Autodesk Inventor part; units mm, degrees
(part 2 of 3)
  line L886 (-89.9741, -91.3777) -> (-89.3883, -91.9634) construction
  line L887 (-89.3883, -91.9634) -> (-88.4384, -91.9634) construction
  line L888 (-88.4384, -91.9634) -> (-87.8528, -91.3777) construction
  line L889 (-87.8528, -91.3777) -> (-82.9029, -86.4278)
  spline S5 degree 3 poles (-82.9029, -86.4278) (-82.3172, -85.8421) (-82.3172, -84.8923) (-82.9029, -84.3067) knots 4 4 4 4 5 5 5 5
  line L890 (-82.9029, -86.4278) -> (-82.3172, -85.8421) construction
  line L891 (-82.3172, -85.8421) -> (-82.3172, -84.8923) construction
  line L892 (-82.3172, -84.8923) -> (-82.9029, -84.3067) construction
  line L893 (-82.9029, -84.3067) -> (-84.3171, -82.8924)
  spline S6 degree 3 poles (-84.3171, -82.8924) (-84.9029, -82.3064) (-85.8527, -82.3064) (-86.4384, -82.8924) knots 6 6 6 6 7 7 7 7
  line L894 (-84.3171, -82.8924) -> (-84.9029, -82.3064) construction
  line L895 (-84.9029, -82.3064) -> (-85.8527, -82.3064) construction
  line L896 (-85.8527, -82.3064) -> (-86.4384, -82.8924) construction
  line L897 (-86.4384, -82.8924) -> (-91.3883, -87.842)
  spline S7 degree 3 poles (-72.0243, -68.4782) (-72.6101, -69.0638) (-72.6101, -70.0136) (-72.0243, -70.5993) knots 0 0 0 0 1 1 1 1
  line L898 (-72.0243, -68.4782) -> (-72.6101, -69.0638) construction
  line L899 (-72.6101, -69.0638) -> (-72.6101, -70.0136) construction
  line L900 (-72.6101, -70.0136) -> (-72.0243, -70.5993) construction
  line L901 (-72.0243, -70.5993) -> (-70.6101, -72.0135)
  spline S8 degree 3 poles (-70.6101, -72.0135) (-70.0242, -72.5995) (-69.0746, -72.5995) (-68.4888, -72.0135) knots 2 2 2 2 3 3 3 3
  line L902 (-70.6101, -72.0135) -> (-70.0242, -72.5995) construction
  line L903 (-70.0242, -72.5995) -> (-69.0746, -72.5995) construction
  line L904 (-69.0746, -72.5995) -> (-68.4888, -72.0135) construction
  line L905 (-68.4888, -72.0135) -> (-63.539, -67.064)
  spline S9 degree 3 poles (-63.539, -67.064) (-62.9532, -66.4779) (-62.9532, -65.5285) (-63.539, -64.9425) knots 4 4 4 4 5 5 5 5
  line L906 (-63.539, -67.064) -> (-62.9532, -66.4779) construction
  line L907 (-62.9532, -66.4779) -> (-62.9532, -65.5285) construction
  line L908 (-62.9532, -65.5285) -> (-63.539, -64.9425) construction
  line L909 (-63.539, -64.9425) -> (-64.9532, -63.5282)
  spline S10 degree 3 poles (-64.9532, -63.5282) (-65.5391, -62.9426) (-66.4887, -62.9426) (-67.0745, -63.5282) knots 6 6 6 6 7 7 7 7
  line L910 (-64.9532, -63.5282) -> (-65.5391, -62.9426) construction
  line L911 (-65.5391, -62.9426) -> (-66.4887, -62.9426) construction
  line L912 (-66.4887, -62.9426) -> (-67.0745, -63.5282) construction
  line L913 (-67.0745, -63.5282) -> (-72.0243, -68.4782)
  spline S11 degree 3 poles (-52.6603, -49.114) (-53.2461, -49.7) (-53.2461, -50.6498) (-52.6603, -51.2355) knots 0 0 0 0 1 1 1 1
  line L914 (-52.6603, -49.114) -> (-53.2461, -49.7) construction
  line L915 (-53.2461, -49.7) -> (-53.2461, -50.6498) construction
  line L916 (-53.2461, -50.6498) -> (-52.6603, -51.2355) construction
  line L917 (-52.6603, -51.2355) -> (-51.2461, -52.6497)
  spline S12 degree 3 poles (-51.2461, -52.6497) (-50.6602, -53.2353) (-49.7106, -53.2353) (-49.1247, -52.6497) knots 2 2 2 2 3 3 3 3
  line L918 (-51.2461, -52.6497) -> (-50.6602, -53.2353) construction
  line L919 (-50.6602, -53.2353) -> (-49.7106, -53.2353) construction
  line L920 (-49.7106, -53.2353) -> (-49.1247, -52.6497) construction
  line L921 (-49.1247, -52.6497) -> (-44.175, -47.6998)
  spline S13 degree 3 poles (-44.175, -47.6998) (-43.5892, -47.1141) (-43.5892, -46.1643) (-44.175, -45.5786) knots 4 4 4 4 5 5 5 5
  line L922 (-44.175, -47.6998) -> (-43.5892, -47.1141) construction
  line L923 (-43.5892, -47.1141) -> (-43.5892, -46.1643) construction
  line L924 (-43.5892, -46.1643) -> (-44.175, -45.5786) construction
  line L925 (-44.175, -45.5786) -> (-45.5892, -44.1644)
  spline S14 degree 3 poles (-45.5892, -44.1644) (-46.175, -43.5787) (-47.1249, -43.5787) (-47.7105, -44.1644) knots 6 6 6 6 7 7 7 7
  line L926 (-45.5892, -44.1644) -> (-46.175, -43.5787) construction
  line L927 (-46.175, -43.5787) -> (-47.1249, -43.5787) construction
  line L928 (-47.1249, -43.5787) -> (-47.7105, -44.1644) construction
  line L929 (-47.7105, -44.1644) -> (-52.6603, -49.114)
  spline S15 degree 3 poles (-33.2964, -29.7501) (-33.8821, -30.3358) (-33.8821, -31.2856) (-33.2964, -31.8716) knots 0 0 0 0 1 1 1 1
  line L930 (-33.2964, -29.7501) -> (-33.8821, -30.3358) construction
  line L931 (-33.8821, -30.3358) -> (-33.8821, -31.2856) construction
  line L932 (-33.8821, -31.2856) -> (-33.2964, -31.8716) construction
  line L933 (-33.2964, -31.8716) -> (-31.8822, -33.2858)
  spline S16 degree 3 poles (-31.8822, -33.2858) (-31.2964, -33.8715) (-30.3466, -33.8715) (-29.7609, -33.2858) knots 2 2 2 2 3 3 3 3
  line L934 (-31.8822, -33.2858) -> (-31.2964, -33.8715) construction
  line L935 (-31.2964, -33.8715) -> (-30.3466, -33.8715) construction
  line L936 (-30.3466, -33.8715) -> (-29.7609, -33.2858) construction
  line L937 (-29.7609, -33.2858) -> (-24.811, -28.3359)
  spline S17 degree 3 poles (-24.811, -28.3359) (-24.2253, -27.7502) (-24.2253, -26.8004) (-24.811, -26.2148) knots 4 4 4 4 5 5 5 5
  line L938 (-24.811, -28.3359) -> (-24.2253, -27.7502) construction
  line L939 (-24.2253, -27.7502) -> (-24.2253, -26.8004) construction
  line L940 (-24.2253, -26.8004) -> (-24.811, -26.2148) construction
  line L941 (-24.811, -26.2148) -> (-26.2252, -24.8006)
  spline S18 degree 3 poles (-26.2252, -24.8006) (-26.811, -24.2145) (-27.7608, -24.2145) (-28.3467, -24.8006) knots 6 6 6 6 7 7 7 7
  line L942 (-26.2252, -24.8006) -> (-26.811, -24.2145) construction
  line L943 (-26.811, -24.2145) -> (-27.7608, -24.2145) construction
  line L944 (-27.7608, -24.2145) -> (-28.3467, -24.8006) construction
  line L945 (-28.3467, -24.8006) -> (-33.2964, -29.7501)
  spline S19 degree 3 poles (-13.9324, -10.3863) (-14.5182, -10.9719) (-14.5182, -11.9218) (-13.9324, -12.5074) knots 0 0 0 0 1 1 1 1
  line L946 (-13.9324, -10.3863) -> (-14.5182, -10.9719) construction
  line L947 (-14.5182, -10.9719) -> (-14.5182, -11.9218) construction
  line L948 (-14.5182, -11.9218) -> (-13.9324, -12.5074) construction
  line L949 (-13.9324, -12.5074) -> (-12.5182, -13.9216)
  spline S20 degree 3 poles (-12.5182, -13.9216) (-11.9323, -14.5076) (-10.9827, -14.5076) (-10.3969, -13.9216) knots 2 2 2 2 3 3 3 3
  line L950 (-12.5182, -13.9216) -> (-11.9323, -14.5076) construction
  line L951 (-11.9323, -14.5076) -> (-10.9827, -14.5076) construction
  line L952 (-10.9827, -14.5076) -> (-10.3969, -13.9216) construction
  line L953 (-10.3969, -13.9216) -> (-5.4471, -8.9721)
  spline S21 degree 3 poles (-5.4471, -8.9721) (-4.8613, -8.3861) (-4.8613, -7.4366) (-5.4471, -6.8506) knots 4 4 4 4 5 5 5 5
  line L954 (-5.4471, -8.9721) -> (-4.8613, -8.3861) construction
  line L955 (-4.8613, -8.3861) -> (-4.8613, -7.4366) construction
  line L956 (-4.8613, -7.4366) -> (-5.4471, -6.8506) construction
  line L957 (-5.4471, -6.8506) -> (-6.8613, -5.4364)
  spline S22 degree 3 poles (-6.8613, -5.4364) (-7.4472, -4.8507) (-8.3968, -4.8507) (-8.9827, -5.4364) knots 6 6 6 6 7 7 7 7
  line L958 (-6.8613, -5.4364) -> (-7.4472, -4.8507) construction
  line L959 (-7.4472, -4.8507) -> (-8.3968, -4.8507) construction
  line L960 (-8.3968, -4.8507) -> (-8.9827, -5.4364) construction
  line L961 (-8.9827, -5.4364) -> (-13.9324, -10.3863)
  spline S23 degree 3 poles (5.4315, 8.9777) (4.8458, 8.3919) (4.8458, 7.4423) (5.4315, 6.8564) knots 0 0 0 0 1 1 1 1
  line L962 (5.4315, 8.9777) -> (4.8458, 8.3919) construction
  line L963 (4.8458, 8.3919) -> (4.8458, 7.4423) construction
  line L964 (4.8458, 7.4423) -> (5.4315, 6.8564) construction
  line L965 (5.4315, 6.8564) -> (6.8457, 5.4422)
  spline S24 degree 3 poles (6.8457, 5.4422) (7.4317, 4.8564) (8.3815, 4.8564) (8.9672, 5.4422) knots 2 2 2 2 3 3 3 3
  line L966 (6.8457, 5.4422) -> (7.4317, 4.8564) construction
  line L967 (7.4317, 4.8564) -> (8.3815, 4.8564) construction
  line L968 (8.3815, 4.8564) -> (8.9672, 5.4422) construction
  line L969 (8.9672, 5.4422) -> (13.9167, 10.392)
  spline S25 degree 3 poles (13.9167, 10.392) (14.5027, 10.9778) (14.5027, 11.9274) (13.9167, 12.5133) knots 4 4 4 4 5 5 5 5
  line L970 (13.9167, 10.392) -> (14.5027, 10.9778) construction
  line L971 (14.5027, 10.9778) -> (14.5027, 11.9274) construction
  line L972 (14.5027, 11.9274) -> (13.9167, 12.5133) construction
  line L973 (13.9167, 12.5133) -> (12.5025, 13.9275)
  spline S26 degree 3 poles (12.5025, 13.9275) (11.9168, 14.5133) (10.967, 14.5133) (10.3814, 13.9275) knots 6 6 6 6 7 7 7 7
  line L974 (12.5025, 13.9275) -> (11.9168, 14.5133) construction
  line L975 (11.9168, 14.5133) -> (10.967, 14.5133) construction
  line L976 (10.967, 14.5133) -> (10.3814, 13.9275) construction
  line L977 (10.3814, 13.9275) -> (5.4315, 8.9777)
  spline S27 degree 3 poles (24.7956, 28.3418) (24.2096, 27.7559) (24.2096, 26.8061) (24.7956, 26.2204) knots 0 0 0 0 1 1 1 1
  line L978 (24.7956, 28.3418) -> (24.2096, 27.7559) construction
  line L979 (24.2096, 27.7559) -> (24.2096, 26.8061) construction
  line L980 (24.2096, 26.8061) -> (24.7956, 26.2204) construction
  line L981 (24.7956, 26.2204) -> (26.2099, 24.8062)
  spline S28 degree 3 poles (26.2099, 24.8062) (26.7955, 24.2204) (27.7453, 24.2204) (28.331, 24.8062) knots 2 2 2 2 3 3 3 3
  line L982 (26.2099, 24.8062) -> (26.7955, 24.2204) construction
  line L983 (26.7955, 24.2204) -> (27.7453, 24.2204) construction
  line L984 (27.7453, 24.2204) -> (28.331, 24.8062) construction
  line L985 (28.331, 24.8062) -> (33.2809, 29.756)
  spline S29 degree 3 poles (33.2809, 29.756) (33.8666, 30.3416) (33.8666, 31.2915) (33.2809, 31.8773) knots 4 4 4 4 5 5 5 5
  line L986 (33.2809, 29.756) -> (33.8666, 30.3416) construction
  line L987 (33.8666, 30.3416) -> (33.8666, 31.2915) construction
  line L988 (33.8666, 31.2915) -> (33.2809, 31.8773) construction
  line L989 (33.2809, 31.8773) -> (31.8667, 33.2915)
  spline S30 degree 3 poles (31.8667, 33.2915) (31.2807, 33.8773) (30.3312, 33.8773) (29.7452, 33.2915) knots 6 6 6 6 7 7 7 7
  line L990 (31.8667, 33.2915) -> (31.2807, 33.8773) construction
  line L991 (31.2807, 33.8773) -> (30.3312, 33.8773) construction
  line L992 (30.3312, 33.8773) -> (29.7452, 33.2915) construction
  line L993 (29.7452, 33.2915) -> (24.7956, 28.3418)
  spline S31 degree 3 poles (44.1595, 47.7056) (43.5738, 47.1199) (43.5738, 46.1701) (44.1595, 45.5843) knots 0 0 0 0 1 1 1 1
  line L994 (44.1595, 47.7056) -> (43.5738, 47.1199) construction
  line L995 (43.5738, 47.1199) -> (43.5738, 46.1701) construction
  line L996 (43.5738, 46.1701) -> (44.1595, 45.5843) construction
  line L997 (44.1595, 45.5843) -> (45.5737, 44.1701)
  spline S32 degree 3 poles (45.5737, 44.1701) (46.1594, 43.5844) (47.1092, 43.5844) (47.6952, 44.1701) knots 2 2 2 2 3 3 3 3
  line L998 (45.5737, 44.1701) -> (46.1594, 43.5844) construction
  line L999 (46.1594, 43.5844) -> (47.1092, 43.5844) construction
  line L1000 (47.1092, 43.5844) -> (47.6952, 44.1701) construction
  line L1001 (47.6952, 44.1701) -> (52.6448, 49.1198)
  spline S33 degree 3 poles (52.6448, 49.1198) (53.2304, 49.7057) (53.2304, 50.6555) (52.6448, 51.2411) knots 4 4 4 4 5 5 5 5
  line L1002 (52.6448, 49.1198) -> (53.2304, 49.7057) construction
  line L1003 (53.2304, 49.7057) -> (53.2304, 50.6555) construction
  line L1004 (53.2304, 50.6555) -> (52.6448, 51.2411) construction
  line L1005 (52.6448, 51.2411) -> (51.2306, 52.6554)
  spline S34 degree 3 poles (51.2306, 52.6554) (50.6449, 53.2412) (49.6951, 53.2412) (49.1094, 52.6554) knots 6 6 6 6 7 7 7 7
  line L1006 (51.2306, 52.6554) -> (50.6449, 53.2412) construction
  line L1007 (50.6449, 53.2412) -> (49.6951, 53.2412) construction
  line L1008 (49.6951, 53.2412) -> (49.1094, 52.6554) construction
  line L1009 (49.1094, 52.6554) -> (44.1595, 47.7056)
  spline S35 degree 3 poles (63.5233, 67.0696) (62.9377, 66.4838) (62.9377, 65.5342) (63.5233, 64.9483) knots 0 0 0 0 1 1 1 1
  line L1010 (63.5233, 67.0696) -> (62.9377, 66.4838) construction
  line L1011 (62.9377, 66.4838) -> (62.9377, 65.5342) construction
  line L1012 (62.9377, 65.5342) -> (63.5233, 64.9483) construction
  line L1013 (63.5233, 64.9483) -> (64.9376, 63.5341)
  spline S36 degree 3 poles (64.9376, 63.5341) (65.5236, 62.9483) (66.4734, 62.9483) (67.059, 63.5341) knots 2 2 2 2 3 3 3 3
  line L1014 (64.9376, 63.5341) -> (65.5236, 62.9483) construction
  line L1015 (65.5236, 62.9483) -> (66.4734, 62.9483) construction
  line L1016 (66.4734, 62.9483) -> (67.059, 63.5341) construction
  line L1017 (67.059, 63.5341) -> (72.0086, 68.4838)
  spline S37 degree 3 poles (72.0086, 68.4838) (72.5946, 69.0697) (72.5946, 70.0193) (72.0086, 70.6052) knots 4 4 4 4 5 5 5 5
  line L1018 (72.0086, 68.4838) -> (72.5946, 69.0697) construction
  line L1019 (72.5946, 69.0697) -> (72.5946, 70.0193) construction
  line L1020 (72.5946, 70.0193) -> (72.0086, 70.6052) construction
  line L1021 (72.0086, 70.6052) -> (70.5944, 72.0194)
  spline S38 degree 3 poles (70.5944, 72.0194) (70.0087, 72.6052) (69.0589, 72.6052) (68.4733, 72.0194) knots 6 6 6 6 7 7 7 7
  line L1022 (70.5944, 72.0194) -> (70.0087, 72.6052) construction
  line L1023 (70.0087, 72.6052) -> (69.0589, 72.6052) construction
  line L1024 (69.0589, 72.6052) -> (68.4733, 72.0194) construction
  line L1025 (68.4733, 72.0194) -> (63.5233, 67.0696)
  spline S39 degree 3 poles (82.8875, 86.4337) (82.3015, 85.8478) (82.3015, 84.898) (82.8875, 84.3123) knots 0 0 0 0 1 1 1 1
  line L1026 (82.8875, 86.4337) -> (82.3015, 85.8478) construction
  line L1027 (82.3015, 85.8478) -> (82.3015, 84.898) construction
  line L1028 (82.3015, 84.898) -> (82.8875, 84.3123) construction
  line L1029 (82.8875, 84.3123) -> (84.3017, 82.8981)
  spline S40 degree 3 poles (84.3017, 82.8981) (84.8874, 82.3123) (85.8372, 82.3123) (86.4229, 82.8981) knots 2 2 2 2 3 3 3 3
  line L1030 (84.3017, 82.8981) -> (84.8874, 82.3123) construction
  line L1031 (84.8874, 82.3123) -> (85.8372, 82.3123) construction
  line L1032 (85.8372, 82.3123) -> (86.4229, 82.8981) construction
  line L1033 (86.4229, 82.8981) -> (91.3728, 87.8479)
  spline S41 degree 3 poles (91.3728, 87.8479) (91.9585, 88.4335) (91.9585, 89.3833) (91.3728, 89.9692) knots 4 4 4 4 5 5 5 5
  line L1034 (91.3728, 87.8479) -> (91.9585, 88.4335) construction
  line L1035 (91.9585, 88.4335) -> (91.9585, 89.3833) construction
  line L1036 (91.9585, 89.3833) -> (91.3728, 89.9692) construction
  line L1037 (91.3728, 89.9692) -> (89.9586, 91.3834)
  spline S42 degree 3 poles (89.9586, 91.3834) (89.3726, 91.9691) (88.4231, 91.9691) (87.8371, 91.3834) knots 6 6 6 6 7 7 7 7
  line L1038 (89.9586, 91.3834) -> (89.3726, 91.9691) construction
  line L1039 (89.3726, 91.9691) -> (88.4231, 91.9691) construction
  line L1040 (88.4231, 91.9691) -> (87.8371, 91.3834) construction
  line L1041 (87.8371, 91.3834) -> (82.8875, 86.4337)
  spline S43 degree 3 poles (-87.8531, 91.3832) (-88.439, 91.9689) (-89.3886, 91.9689) (-89.9744, 91.3832) knots 0 0 0 0 1 1 1 1
  line L1042 (-87.8531, 91.3832) -> (-88.439, 91.9689) construction
  line L1043 (-88.439, 91.9689) -> (-89.3886, 91.9689) construction
  line L1044 (-89.3886, 91.9689) -> (-89.9744, 91.3832) construction
  line L1045 (-89.9744, 91.3832) -> (-91.3887, 89.969)
  spline S44 degree 3 poles (-91.3887, 89.969) (-91.9745, 89.3832) (-91.9745, 88.4334) (-91.3887, 87.8475) knots 2 2 2 2 3 3 3 3
  line L1046 (-91.3887, 89.969) -> (-91.9745, 89.3832) construction
  line L1047 (-91.9745, 89.3832) -> (-91.9745, 88.4334) construction
  line L1048 (-91.9745, 88.4334) -> (-91.3887, 87.8475) construction
  line L1049 (-91.3887, 87.8475) -> (-86.4389, 82.898)
  spline S45 degree 3 poles (-86.4389, 82.898) (-85.8531, 82.3121) (-84.9034, 82.3121) (-84.3176, 82.898) knots 4 4 4 4 5 5 5 5
  line L1050 (-86.4389, 82.898) -> (-85.8531, 82.3121) construction
  line L1051 (-85.8531, 82.3121) -> (-84.9034, 82.3121) construction
  line L1052 (-84.9034, 82.3121) -> (-84.3176, 82.898) construction
  line L1053 (-84.3176, 82.898) -> (-82.9034, 84.3122)
  spline S46 degree 3 poles (-82.9034, 84.3122) (-82.3175, 84.8978) (-82.3175, 85.8476) (-82.9034, 86.4333) knots 6 6 6 6 7 7 7 7
  line L1054 (-82.9034, 84.3122) -> (-82.3175, 84.8978) construction
  line L1055 (-82.3175, 84.8978) -> (-82.3175, 85.8476) construction
  line L1056 (-82.3175, 85.8476) -> (-82.9034, 86.4333) construction
  line L1057 (-82.9034, 86.4333) -> (-87.8531, 91.3832)
  spline S47 degree 3 poles (-68.4891, 72.0192) (-69.0749, 72.605) (-70.0248, 72.605) (-70.6104, 72.0192) knots 0 0 0 0 1 1 1 1
  line L1058 (-68.4891, 72.0192) -> (-69.0749, 72.605) construction
  line L1059 (-69.0749, 72.605) -> (-70.0248, 72.605) construction
  line L1060 (-70.0248, 72.605) -> (-70.6104, 72.0192) construction
  line L1061 (-70.6104, 72.0192) -> (-72.0246, 70.605)
  spline S48 degree 3 poles (-72.0246, 70.605) (-72.6105, 70.0192) (-72.6105, 69.0693) (-72.0246, 68.4837) knots 2 2 2 2 3 3 3 3
  line L1062 (-72.0246, 70.605) -> (-72.6105, 70.0192) construction
  line L1063 (-72.6105, 70.0192) -> (-72.6105, 69.0693) construction
  line L1064 (-72.6105, 69.0693) -> (-72.0246, 68.4837) construction
  line L1065 (-72.0246, 68.4837) -> (-67.0749, 63.5339)
  spline S49 degree 3 poles (-67.0749, 63.5339) (-66.4892, 62.9481) (-65.5394, 62.9481) (-64.9536, 63.5339) knots 4 4 4 4 5 5 5 5
  line L1066 (-67.0749, 63.5339) -> (-66.4892, 62.9481) construction
  line L1067 (-66.4892, 62.9481) -> (-65.5394, 62.9481) construction
  line L1068 (-65.5394, 62.9481) -> (-64.9536, 63.5339) construction
  line L1069 (-64.9536, 63.5339) -> (-63.5394, 64.9481)
  spline S50 degree 3 poles (-63.5394, 64.9481) (-62.9537, 65.534) (-62.9537, 66.4836) (-63.5394, 67.0695) knots 6 6 6 6 7 7 7 7
  line L1070 (-63.5394, 64.9481) -> (-62.9537, 65.534) construction
  line L1071 (-62.9537, 65.534) -> (-62.9537, 66.4836) construction
  line L1072 (-62.9537, 66.4836) -> (-63.5394, 67.0695) construction
  line L1073 (-63.5394, 67.0695) -> (-68.4891, 72.0192)
  spline S51 degree 3 poles (-49.1253, 52.6552) (-49.7109, 53.241) (-50.6607, 53.241) (-51.2466, 52.6552) knots 0 0 0 0 1 1 1 1
  line L1074 (-49.1253, 52.6552) -> (-49.7109, 53.241) construction
  line L1075 (-49.7109, 53.241) -> (-50.6607, 53.241) construction
  line L1076 (-50.6607, 53.241) -> (-51.2466, 52.6552) construction
  line L1077 (-51.2466, 52.6552) -> (-52.6608, 51.241)
  spline S52 degree 3 poles (-52.6608, 51.241) (-53.2464, 50.6553) (-53.2464, 49.7055) (-52.6608, 49.1197) knots 2 2 2 2 3 3 3 3
  line L1078 (-52.6608, 51.241) -> (-53.2464, 50.6553) construction
  line L1079 (-53.2464, 50.6553) -> (-53.2464, 49.7055) construction
  line L1080 (-53.2464, 49.7055) -> (-52.6608, 49.1197) construction
  line L1081 (-52.6608, 49.1197) -> (-47.711, 44.1699)
  spline S53 degree 3 poles (-47.711, 44.1699) (-47.1252, 43.5841) (-46.1754, 43.5841) (-45.5897, 44.1699) knots 4 4 4 4 5 5 5 5
  line L1082 (-47.711, 44.1699) -> (-47.1252, 43.5841) construction
  line L1083 (-47.1252, 43.5841) -> (-46.1754, 43.5841) construction
  line L1084 (-46.1754, 43.5841) -> (-45.5897, 44.1699) construction
  line L1085 (-45.5897, 44.1699) -> (-44.1755, 45.5841)
  spline S54 degree 3 poles (-44.1755, 45.5841) (-43.5897, 46.17) (-43.5897, 47.1196) (-44.1755, 47.7054) knots 6 6 6 6 7 7 7 7
  line L1086 (-44.1755, 45.5841) -> (-43.5897, 46.17) construction
  line L1087 (-43.5897, 46.17) -> (-43.5897, 47.1196) construction
  line L1088 (-43.5897, 47.1196) -> (-44.1755, 47.7054) construction
  line L1089 (-44.1755, 47.7054) -> (-49.1253, 52.6552)
  spline S55 degree 3 poles (-29.7612, 33.2913) (-30.3471, 33.877) (-31.2967, 33.877) (-31.8826, 33.2913) knots 0 0 0 0 1 1 1 1
  line L1090 (-29.7612, 33.2913) -> (-30.3471, 33.877) construction
  line L1091 (-30.3471, 33.877) -> (-31.2967, 33.877) construction
  line L1092 (-31.2967, 33.877) -> (-31.8826, 33.2913) construction
  line L1093 (-31.8826, 33.2913) -> (-33.2968, 31.8771)
  spline S56 degree 3 poles (-33.2968, 31.8771) (-33.8826, 31.2913) (-33.8826, 30.3415) (-33.2968, 29.7556) knots 2 2 2 2 3 3 3 3
  line L1094 (-33.2968, 31.8771) -> (-33.8826, 31.2913) construction
  line L1095 (-33.8826, 31.2913) -> (-33.8826, 30.3415) construction
  line L1096 (-33.8826, 30.3415) -> (-33.2968, 29.7556) construction
  line L1097 (-33.2968, 29.7556) -> (-28.347, 24.8061)
  spline S57 degree 3 poles (-28.347, 24.8061) (-27.7612, 24.2202) (-26.8115, 24.2202) (-26.2257, 24.8061) knots 4 4 4 4 5 5 5 5
  line L1098 (-28.347, 24.8061) -> (-27.7612, 24.2202) construction
  line L1099 (-27.7612, 24.2202) -> (-26.8115, 24.2202) construction
  line L1100 (-26.8115, 24.2202) -> (-26.2257, 24.8061) construction
  line L1101 (-26.2257, 24.8061) -> (-24.8115, 26.2203)
  spline S58 degree 3 poles (-24.8115, 26.2203) (-24.2257, 26.8059) (-24.2257, 27.7558) (-24.8115, 28.3414) knots 6 6 6 6 7 7 7 7
  line L1102 (-24.8115, 26.2203) -> (-24.2257, 26.8059) construction
  line L1103 (-24.2257, 26.8059) -> (-24.2257, 27.7558) construction
  line L1104 (-24.2257, 27.7558) -> (-24.8115, 28.3414) construction
  line L1105 (-24.8115, 28.3414) -> (-29.7612, 33.2913)
  spline S59 degree 3 poles (-10.3972, 13.9273) (-10.9831, 14.5132) (-11.9329, 14.5132) (-12.5185, 13.9273) knots 0 0 0 0 1 1 1 1
  line L1106 (-10.3972, 13.9273) -> (-10.9831, 14.5132) construction
  line L1107 (-10.9831, 14.5132) -> (-11.9329, 14.5132) construction
  line L1108 (-11.9329, 14.5132) -> (-12.5185, 13.9273) construction
  line L1109 (-12.5185, 13.9273) -> (-13.9327, 12.5131)
  spline S60 degree 3 poles (-13.9327, 12.5131) (-14.5186, 11.9273) (-14.5186, 10.9776) (-13.9327, 10.3918) knots 2 2 2 2 3 3 3 3
  line L1110 (-13.9327, 12.5131) -> (-14.5186, 11.9273) construction
  line L1111 (-14.5186, 11.9273) -> (-14.5186, 10.9776) construction
  line L1112 (-14.5186, 10.9776) -> (-13.9327, 10.3918) construction
  line L1113 (-13.9327, 10.3918) -> (-8.983, 5.442)
  spline S61 degree 3 poles (-8.983, 5.442) (-8.3973, 4.8562) (-7.4475, 4.8562) (-6.8617, 5.442) knots 4 4 4 4 5 5 5 5
  line L1114 (-8.983, 5.442) -> (-8.3973, 4.8562) construction
  line L1115 (-8.3973, 4.8562) -> (-7.4475, 4.8562) construction
  line L1116 (-7.4475, 4.8562) -> (-6.8617, 5.442) construction
  line L1117 (-6.8617, 5.442) -> (-5.4475, 6.8563)
  spline S62 degree 3 poles (-5.4475, 6.8563) (-4.8618, 7.4421) (-4.8618, 8.3917) (-5.4475, 8.9776) knots 6 6 6 6 7 7 7 7
  line L1118 (-5.4475, 6.8563) -> (-4.8618, 7.4421) construction
  line L1119 (-4.8618, 7.4421) -> (-4.8618, 8.3917) construction
  line L1120 (-4.8618, 8.3917) -> (-5.4475, 8.9776) construction
  line L1121 (-5.4475, 8.9776) -> (-10.3972, 13.9273)
  spline S63 degree 3 poles (8.9668, -5.4367) (8.3808, -4.851) (7.431, -4.851) (6.8453, -5.4367) knots 0 0 0 0 1 1 1 1
  line L1122 (8.9668, -5.4367) -> (8.3808, -4.851) construction
  line L1123 (8.3808, -4.851) -> (7.431, -4.851) construction
  line L1124 (7.431, -4.851) -> (6.8453, -5.4367) construction
  line L1125 (6.8453, -5.4367) -> (5.4311, -6.8509)
  spline S64 degree 3 poles (5.4311, -6.8509) (4.8454, -7.4366) (4.8454, -8.3864) (5.4311, -8.9721) knots 2 2 2 2 3 3 3 3
  line L1126 (5.4311, -6.8509) -> (4.8454, -7.4366) construction
  line L1127 (4.8454, -7.4366) -> (4.8454, -8.3864) construction
  line L1128 (4.8454, -8.3864) -> (5.4311, -8.9721) construction
  line L1129 (5.4311, -8.9721) -> (10.381, -13.922)
  spline S65 degree 3 poles (10.381, -13.922) (10.9667, -14.5076) (11.9165, -14.5076) (12.5022, -13.922) knots 4 4 4 4 5 5 5 5
  line L1130 (10.381, -13.922) -> (10.9667, -14.5076) construction
  line L1131 (10.9667, -14.5076) -> (11.9165, -14.5076) construction
  line L1132 (11.9165, -14.5076) -> (12.5022, -13.922) construction
  line L1133 (12.5022, -13.922) -> (13.9164, -12.5078)
  spline S66 degree 3 poles (13.9164, -12.5078) (14.502, -11.9221) (14.502, -10.9723) (13.9164, -10.3863) knots 6 6 6 6 7 7 7 7
  line L1134 (13.9164, -12.5078) -> (14.502, -11.9221) construction
  line L1135 (14.502, -11.9221) -> (14.502, -10.9723) construction
  line L1136 (14.502, -10.9723) -> (13.9164, -10.3863) construction
  line L1137 (13.9164, -10.3863) -> (8.9668, -5.4367)
  spline S67 degree 3 poles (28.3307, -24.8006) (27.745, -24.2149) (26.7952, -24.2149) (26.2092, -24.8006) knots 0 0 0 0 1 1 1 1
  line L1138 (28.3307, -24.8006) -> (27.745, -24.2149) construction
  line L1139 (27.745, -24.2149) -> (26.7952, -24.2149) construction
  line L1140 (26.7952, -24.2149) -> (26.2092, -24.8006) construction
  line L1141 (26.2092, -24.8006) -> (24.795, -26.2148)
  spline S68 degree 3 poles (24.795, -26.2148) (24.2093, -26.8008) (24.2093, -27.7502) (24.795, -28.3363) knots 2 2 2 2 3 3 3 3
  line L1142 (24.795, -26.2148) -> (24.2093, -26.8008) construction
  line L1143 (24.2093, -26.8008) -> (24.2093, -27.7502) construction
  line L1144 (24.2093, -27.7502) -> (24.795, -28.3363) construction
  line L1145 (24.795, -28.3363) -> (29.7449, -33.2858)
  spline S69 degree 3 poles (29.7449, -33.2858) (30.3305, -33.8718) (31.2803, -33.8718) (31.866, -33.2858) knots 4 4 4 4 5 5 5 5
  line L1146 (29.7449, -33.2858) -> (30.3305, -33.8718) construction
  line L1147 (30.3305, -33.8718) -> (31.2803, -33.8718) construction
  line L1148 (31.2803, -33.8718) -> (31.866, -33.2858) construction
  line L1149 (31.866, -33.2858) -> (33.2802, -31.8716)
  spline S70 degree 3 poles (33.2802, -31.8716) (33.8662, -31.2859) (33.8662, -30.3361) (33.2802, -29.7505) knots 6 6 6 6 7 7 7 7
  line L1150 (33.2802, -31.8716) -> (33.8662, -31.2859) construction
  line L1151 (33.8662, -31.2859) -> (33.8662, -30.3361) construction
  line L1152 (33.8662, -30.3361) -> (33.2802, -29.7505) construction
  line L1153 (33.2802, -29.7505) -> (28.3307, -24.8006)
  spline S71 degree 3 poles (47.6945, -44.1647) (47.1088, -43.5787) (46.159, -43.5787) (45.5734, -44.1647) knots 0 0 0 0 1 1 1 1
  line L1154 (47.6945, -44.1647) -> (47.1088, -43.5787) construction
  line L1155 (47.1088, -43.5787) -> (46.159, -43.5787) construction
  line L1156 (46.159, -43.5787) -> (45.5734, -44.1647) construction
  line L1157 (45.5734, -44.1647) -> (44.1591, -45.579)
  spline S72 degree 3 poles (44.1591, -45.579) (43.5731, -46.1646) (43.5731, -47.1144) (44.1591, -47.7001) knots 2 2 2 2 3 3 3 3
  line L1158 (44.1591, -45.579) -> (43.5731, -46.1646) construction
  line L1159 (43.5731, -46.1646) -> (43.5731, -47.1144) construction
  line L1160 (43.5731, -47.1144) -> (44.1591, -47.7001) construction
  line L1161 (44.1591, -47.7001) -> (49.1087, -52.65)
  spline S73 degree 3 poles (49.1087, -52.65) (49.6947, -53.2357) (50.6442, -53.2357) (51.2302, -52.65) knots 4 4 4 4 5 5 5 5
  line L1162 (49.1087, -52.65) -> (49.6947, -53.2357) construction
  line L1163 (49.6947, -53.2357) -> (50.6442, -53.2357) construction
  line L1164 (50.6442, -53.2357) -> (51.2302, -52.65) construction
  line L1165 (51.2302, -52.65) -> (52.6444, -51.2358)
  spline S74 degree 3 poles (52.6444, -51.2358) (53.2301, -50.6498) (53.2301, -49.7) (52.6444, -49.1143) knots 6 6 6 6 7 7 7 7
  line L1166 (52.6444, -51.2358) -> (53.2301, -50.6498) construction
  line L1167 (53.2301, -50.6498) -> (53.2301, -49.7) construction
  line L1168 (53.2301, -49.7) -> (52.6444, -49.1143) construction
  line L1169 (52.6444, -49.1143) -> (47.6945, -44.1647)
  spline S75 degree 3 poles (67.0587, -63.5286) (66.4727, -62.9429) (65.5229, -62.9429) (64.9372, -63.5286) knots 0 0 0 0 1 1 1 1
  line L1170 (67.0587, -63.5286) -> (66.4727, -62.9429) construction
  line L1171 (66.4727, -62.9429) -> (65.5229, -62.9429) construction
  line L1172 (65.5229, -62.9429) -> (64.9372, -63.5286) construction
  line L1173 (64.9372, -63.5286) -> (63.523, -64.9428)
  spline S76 degree 3 poles (63.523, -64.9428) (62.9373, -65.5285) (62.9373, -66.4783) (63.523, -67.064) knots 2 2 2 2 3 3 3 3
  line L1174 (63.523, -64.9428) -> (62.9373, -65.5285) construction
  line L1175 (62.9373, -65.5285) -> (62.9373, -66.4783) construction
  line L1176 (62.9373, -66.4783) -> (63.523, -67.064) construction
  line L1177 (63.523, -67.064) -> (68.4729, -72.0139)
  spline S77 degree 3 poles (68.4729, -72.0139) (69.0586, -72.5995) (70.0084, -72.5995) (70.5941, -72.0139) knots 4 4 4 4 5 5 5 5
  line L1178 (68.4729, -72.0139) -> (69.0586, -72.5995) construction
  line L1179 (69.0586, -72.5995) -> (70.0084, -72.5995) construction
  line L1180 (70.0084, -72.5995) -> (70.5941, -72.0139) construction
  line L1181 (70.5941, -72.0139) -> (72.0083, -70.5997)
  spline S78 degree 3 poles (72.0083, -70.5997) (72.5939, -70.014) (72.5939, -69.0642) (72.0083, -68.4782) knots 6 6 6 6 7 7 7 7
  line L1182 (72.0083, -70.5997) -> (72.5939, -70.014) construction
  line L1183 (72.5939, -70.014) -> (72.5939, -69.0642) construction
  line L1184 (72.5939, -69.0642) -> (72.0083, -68.4782) construction
  line L1185 (72.0083, -68.4782) -> (67.0587, -63.5286)
  spline S79 degree 3 poles (86.4225, -82.8924) (85.8369, -82.3068) (84.8871, -82.3068) (84.3011, -82.8924) knots 0 0 0 0 1 1 1 1
  line L1186 (86.4225, -82.8924) -> (85.8369, -82.3068) construction
  line L1187 (85.8369, -82.3068) -> (84.8871, -82.3068) construction
  line L1188 (84.8871, -82.3068) -> (84.3011, -82.8924) construction
  line L1189 (84.3011, -82.8924) -> (82.8868, -84.3067)
  spline S80 degree 3 poles (82.8868, -84.3067) (82.3012, -84.8927) (82.3012, -85.8421) (82.8868, -86.4281) knots 2 2 2 2 3 3 3 3
  line L1190 (82.8868, -84.3067) -> (82.3012, -84.8927) construction
  line L1191 (82.3012, -84.8927) -> (82.3012, -85.8421) construction
  line L1192 (82.3012, -85.8421) -> (82.8868, -86.4281) construction
  line L1193 (82.8868, -86.4281) -> (87.8368, -91.3777)
  spline S81 degree 3 poles (87.8368, -91.3777) (88.4224, -91.9637) (89.3722, -91.9637) (89.9579, -91.3777) knots 4 4 4 4 5 5 5 5
  line L1194 (87.8368, -91.3777) -> (88.4224, -91.9637) construction
  line L1195 (88.4224, -91.9637) -> (89.3722, -91.9637) construction
  line L1196 (89.3722, -91.9637) -> (89.9579, -91.3777) construction
  line L1197 (89.9579, -91.3777) -> (91.3721, -89.9635)
  spline S82 degree 3 poles (91.3721, -89.9635) (91.9581, -89.3778) (91.9581, -88.428) (91.3721, -87.8424) knots 6 6 6 6 7 7 7 7
  line L1198 (91.3721, -89.9635) -> (91.9581, -89.3778) construction
  line L1199 (91.9581, -89.3778) -> (91.9581, -88.428) construction
  line L1200 (91.9581, -88.428) -> (91.3721, -87.8424) construction
  line L1201 (91.3721, -87.8424) -> (86.4225, -82.8924)
  spline S83 degree 3 poles (-63.5016, -23.5052) (-63.5016, -24.3337) (-62.83, -25.0052) (-62.0016, -25.0052) knots 0 0 0 0 1 1 1 1
  line L1202 (-63.5016, -23.5052) -> (-63.5016, -24.3337) construction
  line L1203 (-63.5016, -24.3337) -> (-62.83, -25.0052) construction
  line L1204 (-62.83, -25.0052) -> (-62.0016, -25.0052) construction
  line L1205 (-62.0016, -25.0052) -> (-60.0016, -25.0052)
  spline S84 degree 3 poles (-60.0016, -25.0052) (-59.1732, -25.0052) (-58.5016, -24.3337) (-58.5016, -23.5052) knots 2 2 2 2 3 3 3 3
  line L1206 (-60.0016, -25.0052) -> (-59.1732, -25.0052) construction
  line L1207 (-59.1732, -25.0052) -> (-58.5016, -24.3337) construction
  line L1208 (-58.5016, -24.3337) -> (-58.5016, -23.5052) construction
  line L1209 (-58.5016, -23.5052) -> (-58.5016, -16.5055)
  spline S85 degree 3 poles (-58.5016, -16.5055) (-58.5016, -15.6769) (-59.1732, -15.0055) (-60.0016, -15.0055) knots 4 4 4 4 5 5 5 5
  line L1210 (-58.5016, -16.5055) -> (-58.5016, -15.6769) construction
  line L1211 (-58.5016, -15.6769) -> (-59.1732, -15.0055) construction
  line L1212 (-59.1732, -15.0055) -> (-60.0016, -15.0055) construction
  line L1213 (-60.0016, -15.0055) -> (-62.0016, -15.0055)
  spline S86 degree 3 poles (-62.0016, -15.0055) (-62.83, -15.0055) (-63.5016, -15.6769) (-63.5016, -16.5055) knots 6 6 6 6 7 7 7 7
  line L1214 (-62.0016, -15.0055) -> (-62.83, -15.0055) construction
  line L1215 (-62.83, -15.0055) -> (-63.5016, -15.6769) construction
  line L1216 (-63.5016, -15.6769) -> (-63.5016, -16.5055) construction
  line L1217 (-63.5016, -16.5055) -> (-63.5016, -23.5052)
  spline S87 degree 3 poles (-63.5016, -3.5054) (-63.5016, -4.3339) (-62.83, -5.0054) (-62.0016, -5.0054) knots 0 0 0 0 1 1 1 1
  line L1218 (-63.5016, -3.5054) -> (-63.5016, -4.3339) construction
  line L1219 (-63.5016, -4.3339) -> (-62.83, -5.0054) construction
  line L1220 (-62.83, -5.0054) -> (-62.0016, -5.0054) construction
  line L1221 (-62.0016, -5.0054) -> (-60.0016, -5.0054)
  spline S88 degree 3 poles (-60.0016, -5.0054) (-59.1732, -5.0054) (-58.5016, -4.3339) (-58.5016, -3.5054) knots 2 2 2 2 3 3 3 3
  line L1222 (-60.0016, -5.0054) -> (-59.1732, -5.0054) construction
  line L1223 (-59.1732, -5.0054) -> (-58.5016, -4.3339) construction
  line L1224 (-58.5016, -4.3339) -> (-58.5016, -3.5054) construction
  line L1225 (-58.5016, -3.5054) -> (-58.5016, 3.4947)
  spline S89 degree 3 poles (-58.5016, 3.4947) (-58.5016, 4.3231) (-59.1732, 4.9947) (-60.0016, 4.9947) knots 4 4 4 4 5 5 5 5
  line L1226 (-58.5016, 3.4947) -> (-58.5016, 4.3231) construction
  line L1227 (-58.5016, 4.3231) -> (-59.1732, 4.9947) construction
  line L1228 (-59.1732, 4.9947) -> (-60.0016, 4.9947) construction
  line L1229 (-60.0016, 4.9947) -> (-62.0016, 4.9947)
  spline S90 degree 3 poles (-62.0016, 4.9947) (-62.83, 4.9947) (-63.5016, 4.3231) (-63.5016, 3.4947) knots 6 6 6 6 7 7 7 7
  line L1230 (-62.0016, 4.9947) -> (-62.83, 4.9947) construction
  line L1231 (-62.83, 4.9947) -> (-63.5016, 4.3231) construction
  line L1232 (-63.5016, 4.3231) -> (-63.5016, 3.4947) construction
  line L1233 (-63.5016, 3.4947) -> (-63.5016, -3.5054)
  spline S91 degree 3 poles (-63.5016, 16.4946) (-63.5016, 15.6662) (-62.83, 14.9946) (-62.0016, 14.9946) knots 0 0 0 0 1 1 1 1
  line L1234 (-63.5016, 16.4946) -> (-63.5016, 15.6662) construction
  line L1235 (-63.5016, 15.6662) -> (-62.83, 14.9946) construction
  line L1236 (-62.83, 14.9946) -> (-62.0016, 14.9946) construction
  line L1237 (-62.0016, 14.9946) -> (-60.0016, 14.9946)
  spline S92 degree 3 poles (-60.0016, 14.9946) (-59.1732, 14.9946) (-58.5016, 15.6662) (-58.5016, 16.4946) knots 2 2 2 2 3 3 3 3
  line L1238 (-60.0016, 14.9946) -> (-59.1732, 14.9946) construction
  line L1239 (-59.1732, 14.9946) -> (-58.5016, 15.6662) construction
  line L1240 (-58.5016, 15.6662) -> (-58.5016, 16.4946) construction
  line L1241 (-58.5016, 16.4946) -> (-58.5016, 23.4947)
  spline S93 degree 3 poles (-58.5016, 23.4947) (-58.5016, 24.3231) (-59.1732, 24.9947) (-60.0016, 24.9947) knots 4 4 4 4 5 5 5 5
  line L1242 (-58.5016, 23.4947) -> (-58.5016, 24.3231) construction
  line L1243 (-58.5016, 24.3231) -> (-59.1732, 24.9947) construction
  line L1244 (-59.1732, 24.9947) -> (-60.0016, 24.9947) construction
  line L1245 (-60.0016, 24.9947) -> (-62.0016, 24.9947)
  spline S94 degree 3 poles (-62.0016, 24.9947) (-62.83, 24.9947) (-63.5016, 24.3231) (-63.5016, 23.4947) knots 6 6 6 6 7 7 7 7
  line L1246 (-62.0016, 24.9947) -> (-62.83, 24.9947) construction
  line L1247 (-62.83, 24.9947) -> (-63.5016, 24.3231) construction
  line L1248 (-63.5016, 24.3231) -> (-63.5016, 23.4947) construction
  line L1249 (-63.5016, 23.4947) -> (-63.5016, 16.4946)
  line L1250 (-65.754, -37.4971) -> (-65.7296, -37.0113)
  line L1251 (-65.7296, -37.0113) -> (-65.6576, -36.5397)
  line L1252 (-65.6576, -36.5397) -> (-65.5406, -36.0846)
  line L1253 (-65.5406, -36.0846) -> (-65.3808, -35.6481)
  line L1254 (-65.3808, -35.6481) -> (-65.1808, -35.233)
  line L1255 (-65.1808, -35.233) -> (-64.9429, -34.8413)
  line L1256 (-64.9429, -34.8413) -> (-64.6694, -34.4754)
  line L1257 (-64.6694, -34.4754) -> (-64.3629, -34.1381)
  line L1258 (-64.3629, -34.1381) -> (-64.0255, -33.8315)
  line L1259 (-64.0255, -33.8315) -> (-63.6599, -33.5583)
  line L1260 (-63.6599, -33.5583) -> (-63.2682, -33.3203)
  line L1261 (-63.2682, -33.3203) -> (-62.8529, -33.1201)
  line L1262 (-62.8529, -33.1201) -> (-62.4166, -32.9606)
  line L1263 (-62.4166, -32.9606) -> (-61.9613, -32.8435)
  line L1264 (-61.9613, -32.8435) -> (-61.4897, -32.7715)
  line L1265 (-61.4897, -32.7715) -> (-61.0041, -32.747)
  line L1266 (-61.0041, -32.747) -> (-60.5184, -32.7715)
  line L1267 (-60.5184, -32.7715) -> (-60.0467, -32.8435)
  line L1268 (-60.0467, -32.8435) -> (-59.5916, -32.9606)
  line L1269 (-59.5916, -32.9606) -> (-59.1551, -33.1201)
  line L1270 (-59.1551, -33.1201) -> (-58.74, -33.3203)
  line L1271 (-58.74, -33.3203) -> (-58.3483, -33.5583)
  line L1272 (-58.3483, -33.5583) -> (-57.9826, -33.8315)
  line L1273 (-57.9826, -33.8315) -> (-57.6453, -34.1381)
  line L1274 (-57.6453, -34.1381) -> (-57.3387, -34.4754)
  line L1275 (-57.3387, -34.4754) -> (-57.0653, -34.8413)
  line L1276 (-57.0653, -34.8413) -> (-56.8275, -35.233)
  line L1277 (-56.8275, -35.233) -> (-56.6273, -35.6481)
  line L1278 (-56.6273, -35.6481) -> (-56.4676, -36.0846)
  line L1279 (-56.4676, -36.0846) -> (-56.3507, -36.5397)
  line L1280 (-56.3507, -36.5397) -> (-56.2786, -37.0113)
  line L1281 (-56.2786, -37.0113) -> (-56.254, -37.4971)
  line L1282 (-56.254, -37.4971) -> (-56.2786, -37.9825)
  line L1283 (-56.2786, -37.9825) -> (-56.3507, -38.4542)
  line L1284 (-56.3507, -38.4542) -> (-56.4676, -38.9096)
  line L1285 (-56.4676, -38.9096) -> (-56.6273, -39.3457)
  line L1286 (-56.6273, -39.3457) -> (-56.8275, -39.7612)
  line L1287 (-56.8275, -39.7612) -> (-57.0653, -40.1529)
  line L1288 (-57.0653, -40.1529) -> (-57.3387, -40.5185)
  line L1289 (-57.3387, -40.5185) -> (-57.6453, -40.8557)
  line L1290 (-57.6453, -40.8557) -> (-57.9826, -41.1623)
  line L1291 (-57.9826, -41.1623) -> (-58.3483, -41.4359)
  line L1292 (-58.3483, -41.4359) -> (-58.74, -41.6736)
  line L1293 (-58.74, -41.6736) -> (-59.1551, -41.8738)
  line L1294 (-59.1551, -41.8738) -> (-59.5916, -42.0336)
  line L1295 (-59.5916, -42.0336) -> (-60.0467, -42.1504)
  line L1296 (-60.0467, -42.1504) -> (-60.5184, -42.2224)
  line L1297 (-60.5184, -42.2224) -> (-61.0041, -42.2469)
  line L1298 (-61.0041, -42.2469) -> (-61.4897, -42.2224)
  line L1299 (-61.4897, -42.2224) -> (-61.9613, -42.1504)
  line L1300 (-61.9613, -42.1504) -> (-62.4166, -42.0336)
  line L1301 (-62.4166, -42.0336) -> (-62.8529, -41.8738)
  line L1302 (-62.8529, -41.8738) -> (-63.2682, -41.6736)
  line L1303 (-63.2682, -41.6736) -> (-63.6599, -41.4359)
  line L1304 (-63.6599, -41.4359) -> (-64.0255, -41.1623)
  line L1305 (-64.0255, -41.1623) -> (-64.3629, -40.8557)
  line L1306 (-64.3629, -40.8557) -> (-64.6694, -40.5185)
  line L1307 (-64.6694, -40.5185) -> (-64.9429, -40.1529)
  line L1308 (-64.9429, -40.1529) -> (-65.1808, -39.7612)
  line L1309 (-65.1808, -39.7612) -> (-65.3808, -39.3457)
  line L1310 (-65.3808, -39.3457) -> (-65.5406, -38.9096)
  line L1311 (-65.5406, -38.9096) -> (-65.6576, -38.4542)
  line L1312 (-65.6576, -38.4542) -> (-65.7296, -37.9825)
  line L1313 (-65.7296, -37.9825) -> (-65.754, -37.4971)
  spline S95 degree 3 poles (57.9681, -23.5052) (57.9681, -24.3337) (58.6396, -25.0052) (59.4681, -25.0052) knots 0 0 0 0 1 1 1 1
  line L1314 (57.9681, -23.5052) -> (57.9681, -24.3337) construction
  line L1315 (57.9681, -24.3337) -> (58.6396, -25.0052) construction
  line L1316 (58.6396, -25.0052) -> (59.4681, -25.0052) construction
  line L1317 (59.4681, -25.0052) -> (61.468, -25.0052)
  spline S96 degree 3 poles (61.468, -25.0052) (62.2965, -25.0052) (62.968, -24.3337) (62.968, -23.5052) knots 2 2 2 2 3 3 3 3
  line L1318 (61.468, -25.0052) -> (62.2965, -25.0052) construction
  line L1319 (62.2965, -25.0052) -> (62.968, -24.3337) construction
  line L1320 (62.968, -24.3337) -> (62.968, -23.5052) construction
  line L1321 (62.968, -23.5052) -> (62.968, -16.5055)
  spline S97 degree 3 poles (62.968, -16.5055) (62.968, -15.6769) (62.2965, -15.0055) (61.468, -15.0055) knots 4 4 4 4 5 5 5 5
  line L1322 (62.968, -16.5055) -> (62.968, -15.6769) construction
  line L1323 (62.968, -15.6769) -> (62.2965, -15.0055) construction
  line L1324 (62.2965, -15.0055) -> (61.468, -15.0055) construction
  line L1325 (61.468, -15.0055) -> (59.4681, -15.0055)
  spline S98 degree 3 poles (59.4681, -15.0055) (58.6396, -15.0055) (57.9681, -15.6769) (57.9681, -16.5055) knots 6 6 6 6 7 7 7 7
  line L1326 (59.4681, -15.0055) -> (58.6396, -15.0055) construction
  line L1327 (58.6396, -15.0055) -> (57.9681, -15.6769) construction
  line L1328 (57.9681, -15.6769) -> (57.9681, -16.5055) construction
  line L1329 (57.9681, -16.5055) -> (57.9681, -23.5052)
  spline S99 degree 3 poles (57.9681, -3.5054) (57.9681, -4.3339) (58.6396, -5.0054) (59.4681, -5.0054) knots 0 0 0 0 1 1 1 1
  line L1330 (57.9681, -3.5054) -> (57.9681, -4.3339) construction
  line L1331 (57.9681, -4.3339) -> (58.6396, -5.0054) construction
  line L1332 (58.6396, -5.0054) -> (59.4681, -5.0054) construction
  line L1333 (59.4681, -5.0054) -> (61.468, -5.0054)
  spline S100 degree 3 poles (61.468, -5.0054) (62.2965, -5.0054) (62.968, -4.3339) (62.968, -3.5054) knots 2 2 2 2 3 3 3 3
  line L1334 (61.468, -5.0054) -> (62.2965, -5.0054) construction
  line L1335 (62.2965, -5.0054) -> (62.968, -4.3339) construction
  line L1336 (62.968, -4.3339) -> (62.968, -3.5054) construction
  line L1337 (62.968, -3.5054) -> (62.968, 3.4947)
  spline S101 degree 3 poles (62.968, 3.4947) (62.968, 4.3231) (62.2965, 4.9947) (61.468, 4.9947) knots 4 4 4 4 5 5 5 5
  line L1338 (62.968, 3.4947) -> (62.968, 4.3231) construction
  line L1339 (62.968, 4.3231) -> (62.2965, 4.9947) construction
  line L1340 (62.2965, 4.9947) -> (61.468, 4.9947) construction
  line L1341 (61.468, 4.9947) -> (59.4681, 4.9947)
  spline S102 degree 3 poles (59.4681, 4.9947) (58.6396, 4.9947) (57.9681, 4.3231) (57.9681, 3.4947) knots 6 6 6 6 7 7 7 7
  line L1342 (59.4681, 4.9947) -> (58.6396, 4.9947) construction
  line L1343 (58.6396, 4.9947) -> (57.9681, 4.3231) construction
  line L1344 (57.9681, 4.3231) -> (57.9681, 3.4947) construction
  line L1345 (57.9681, 3.4947) -> (57.9681, -3.5054)
  spline S103 degree 3 poles (57.9681, 16.4946) (57.9681, 15.6662) (58.6396, 14.9946) (59.4681, 14.9946) knots 0 0 0 0 1 1 1 1
  line L1346 (57.9681, 16.4946) -> (57.9681, 15.6662) construction
  line L1347 (57.9681, 15.6662) -> (58.6396, 14.9946) construction
  line L1348 (58.6396, 14.9946) -> (59.4681, 14.9946) construction
  line L1349 (59.4681, 14.9946) -> (61.468, 14.9946)
  spline S104 degree 3 poles (61.468, 14.9946) (62.2965, 14.9946) (62.968, 15.6662) (62.968, 16.4946) knots 2 2 2 2 3 3 3 3
  line L1350 (61.468, 14.9946) -> (62.2965, 14.9946) construction
  line L1351 (62.2965, 14.9946) -> (62.968, 15.6662) construction
  line L1352 (62.968, 15.6662) -> (62.968, 16.4946) construction
  line L1353 (62.968, 16.4946) -> (62.968, 23.4947)
  spline S105 degree 3 poles (62.968, 23.4947) (62.968, 24.3231) (62.2965, 24.9947) (61.468, 24.9947) knots 4 4 4 4 5 5 5 5
  line L1354 (62.968, 23.4947) -> (62.968, 24.3231) construction
  line L1355 (62.968, 24.3231) -> (62.2965, 24.9947) construction
  line L1356 (62.2965, 24.9947) -> (61.468, 24.9947) construction
  line L1357 (61.468, 24.9947) -> (59.4681, 24.9947)
  spline S106 degree 3 poles (59.4681, 24.9947) (58.6396, 24.9947) (57.9681, 24.3231) (57.9681, 23.4947) knots 6 6 6 6 7 7 7 7
  line L1358 (59.4681, 24.9947) -> (58.6396, 24.9947) construction
  line L1359 (58.6396, 24.9947) -> (57.9681, 24.3231) construction
  line L1360 (57.9681, 24.3231) -> (57.9681, 23.4947) construction
  line L1361 (57.9681, 23.4947) -> (57.9681, 16.4946)
  line L1362 (56.2501, -37.4992) -> (56.2745, -37.0134)
  line L1363 (56.2745, -37.0134) -> (56.3465, -36.5418)
  line L1364 (56.3465, -36.5418) -> (56.4633, -36.0863)
  line L1365 (56.4633, -36.0863) -> (56.6232, -35.6502)
  line L1366 (56.6232, -35.6502) -> (56.8233, -35.2347)
  line L1367 (56.8233, -35.2347) -> (57.061, -34.8434)
  line L1368 (57.061, -34.8434) -> (57.3346, -34.4775)
  line L1369 (57.3346, -34.4775) -> (57.6412, -34.1402)
  line L1370 (57.6412, -34.1402) -> (57.9785, -33.8336)
  line L1371 (57.9785, -33.8336) -> (58.344, -33.5601)
  line L1372 (58.344, -33.5601) -> (58.7357, -33.3223)
  line L1373 (58.7357, -33.3223) -> (59.1508, -33.1222)
  line L1374 (59.1508, -33.1222) -> (59.5873, -32.9627)
  line L1375 (59.5873, -32.9627) -> (60.0428, -32.8455)
  line L1376 (60.0428, -32.8455) -> (60.5144, -32.7735)
  line L1377 (60.5144, -32.7735) -> (60.9998, -32.7491)
  line L1378 (60.9998, -32.7491) -> (61.4856, -32.7735)
  line L1379 (61.4856, -32.7735) -> (61.9572, -32.8455)
  line L1380 (61.9572, -32.8455) -> (62.4123, -32.9627)
  line L1381 (62.4123, -32.9627) -> (62.8488, -33.1222)
  line L1382 (62.8488, -33.1222) -> (63.2639, -33.3223)
  line L1383 (63.2639, -33.3223) -> (63.6556, -33.5601)
  line L1384 (63.6556, -33.5601) -> (64.0215, -33.8336)
  line L1385 (64.0215, -33.8336) -> (64.3588, -34.1402)
  line L1386 (64.3588, -34.1402) -> (64.6654, -34.4775)
  line L1387 (64.6654, -34.4775) -> (64.9386, -34.8434)
  line L1388 (64.9386, -34.8434) -> (65.1766, -35.2347)
  line L1389 (65.1766, -35.2347) -> (65.3768, -35.6502)
  line L1390 (65.3768, -35.6502) -> (65.5363, -36.0863)
  line L1391 (65.5363, -36.0863) -> (65.6534, -36.5418)
  line L1392 (65.6534, -36.5418) -> (65.7254, -37.0134)
  line L1393 (65.7254, -37.0134) -> (65.7499, -37.4992)
  line L1394 (65.7499, -37.4992) -> (65.7254, -37.9846)
  line L1395 (65.7254, -37.9846) -> (65.6534, -38.4562)
  line L1396 (65.6534, -38.4562) -> (65.5363, -38.9117)
  line L1397 (65.5363, -38.9117) -> (65.3768, -39.3478)
  line L1398 (65.3768, -39.3478) -> (65.1766, -39.7633)
  line L1399 (65.1766, -39.7633) -> (64.9386, -40.1547)
  line L1400 (64.9386, -40.1547) -> (64.6654, -40.5205)
  line L1401 (64.6654, -40.5205) -> (64.3588, -40.8578)
  line L1402 (64.3588, -40.8578) -> (64.0215, -41.1644)
  line L1403 (64.0215, -41.1644) -> (63.6556, -41.4376)
  line L1404 (63.6556, -41.4376) -> (63.2639, -41.6757)
  line L1405 (63.2639, -41.6757) -> (62.8488, -41.8758)
  line L1406 (62.8488, -41.8758) -> (62.4123, -42.0353)
  line L1407 (62.4123, -42.0353) -> (61.9572, -42.1525)
  line L1408 (61.9572, -42.1525) -> (61.4856, -42.2245)
  line L1409 (61.4856, -42.2245) -> (60.9998, -42.2489)
  line L1410 (60.9998, -42.2489) -> (60.5144, -42.2245)
  line L1411 (60.5144, -42.2245) -> (60.0428, -42.1525)
  line L1412 (60.0428, -42.1525) -> (59.5873, -42.0353)
  line L1413 (59.5873, -42.0353) -> (59.1508, -41.8758)
  line L1414 (59.1508, -41.8758) -> (58.7357, -41.6757)
  line L1415 (58.7357, -41.6757) -> (58.344, -41.4376)
  line L1416 (58.344, -41.4376) -> (57.9785, -41.1644)
  line L1417 (57.9785, -41.1644) -> (57.6412, -40.8578)
  line L1418 (57.6412, -40.8578) -> (57.3346, -40.5205)
  line L1419 (57.3346, -40.5205) -> (57.061, -40.1547)
  line L1420 (57.061, -40.1547) -> (56.8233, -39.7633)
  line L1421 (56.8233, -39.7633) -> (56.6232, -39.3478)
  line L1422 (56.6232, -39.3478) -> (56.4633, -38.9117)
  line L1423 (56.4633, -38.9117) -> (56.3465, -38.4562)
  line L1424 (56.3465, -38.4562) -> (56.2745, -37.9846)
  line L1425 (56.2745, -37.9846) -> (56.2501, -37.4992)
  line L1426 (56.2459, 37.5119) -> (56.2704, 37.9977)
  line L1427 (56.2704, 37.9977) -> (56.3424, 38.4693)
  line L1428 (56.3424, 38.4693) -> (56.4595, 38.9244)
  line L1429 (56.4595, 38.9244) -> (56.6194, 39.3609)
  line L1430 (56.6194, 39.3609) -> (56.8192, 39.776)
  line L1431 (56.8192, 39.776) -> (57.0572, 40.1677)
  line L1432 (57.0572, 40.1677) -> (57.3304, 40.5334)
  line L1433 (57.3304, 40.5334) -> (57.6371, 40.8707)
  line L1434 (57.6371, 40.8707) -> (57.9743, 41.1773)
  line L1435 (57.9743, 41.1773) -> (58.3402, 41.4507)
  line L1436 (58.3402, 41.4507) -> (58.7319, 41.6888)
  line L1437 (58.7319, 41.6888) -> (59.147, 41.8887)
  line L1438 (59.147, 41.8887) -> (59.5835, 42.0484)
  line L1439 (59.5835, 42.0484) -> (60.0386, 42.1656)
  line L1440 (60.0386, 42.1656) -> (60.5103, 42.2376)
  line L1441 (60.5103, 42.2376) -> (60.996, 42.262)
  line L1442 (60.996, 42.262) -> (61.4814, 42.2376)
  line L1443 (61.4814, 42.2376) -> (61.9531, 42.1656)
  line L1444 (61.9531, 42.1656) -> (62.4085, 42.0484)
  line L1445 (62.4085, 42.0484) -> (62.8447, 41.8887)
  line L1446 (62.8447, 41.8887) -> (63.2601, 41.6888)
  line L1447 (63.2601, 41.6888) -> (63.6518, 41.4507)
  line L1448 (63.6518, 41.4507) -> (64.0174, 41.1773)
  line L1449 (64.0174, 41.1773) -> (64.3546, 40.8707)
  line L1450 (64.3546, 40.8707) -> (64.6613, 40.5334)
  line L1451 (64.6613, 40.5334) -> (64.9348, 40.1677)
  line L1452 (64.9348, 40.1677) -> (65.1725, 39.776)
  line L1453 (65.1725, 39.776) -> (65.3727, 39.3609)
  line L1454 (65.3727, 39.3609) -> (65.5325, 38.9244)
  line L1455 (65.5325, 38.9244) -> (65.6493, 38.4693)
  line L1456 (65.6493, 38.4693) -> (65.7213, 37.9977)
  line L1457 (65.7213, 37.9977) -> (65.7458, 37.5119)
  line L1458 (65.7458, 37.5119) -> (65.7213, 37.0263)
  line L1459 (65.7213, 37.0263) -> (65.6493, 36.5547)
  line L1460 (65.6493, 36.5547) -> (65.5325, 36.0994)
  line L1461 (65.5325, 36.0994) -> (65.3727, 35.6631)
  line L1462 (65.3727, 35.6631) -> (65.1725, 35.2478)
  line L1463 (65.1725, 35.2478) -> (64.9348, 34.8563)
  line L1464 (64.9348, 34.8563) -> (64.6613, 34.4906)
  line L1465 (64.6613, 34.4906) -> (64.3546, 34.1533)
  line L1466 (64.3546, 34.1533) -> (64.0174, 33.8467)
  line L1467 (64.0174, 33.8467) -> (63.6518, 33.5731)
  line L1468 (63.6518, 33.5731) -> (63.2601, 33.3353)
  line L1469 (63.2601, 33.3353) -> (62.8447, 33.1353)
  line L1470 (62.8447, 33.1353) -> (62.4085, 32.9756)
  line L1471 (62.4085, 32.9756) -> (61.9531, 32.8585)
  line L1472 (61.9531, 32.8585) -> (61.4814, 32.7865)
  line L1473 (61.4814, 32.7865) -> (60.996, 32.762)
  line L1474 (60.996, 32.762) -> (60.5103, 32.7865)
  line L1475 (60.5103, 32.7865) -> (60.0386, 32.8585)
  line L1476 (60.0386, 32.8585) -> (59.5835, 32.9756)
  line L1477 (59.5835, 32.9756) -> (59.147, 33.1353)
  line L1478 (59.147, 33.1353) -> (58.7319, 33.3353)
  line L1479 (58.7319, 33.3353) -> (58.3402, 33.5731)
  line L1480 (58.3402, 33.5731) -> (57.9743, 33.8467)